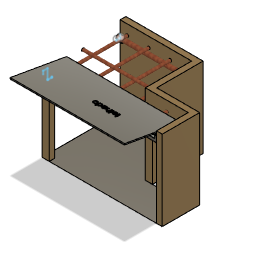
pergolado (Autodesk Fusion 360 design; units mm, degrees)
Autodesk Fusion 360 part; units mm, degrees
note: some values were not read from the file. Set by a fixed rule: which sketch regions a step uses.
sketch "Sketch1" plane through (0, 0, 0) normal (0, 1, 0) x (1, 0, 0)
  line L0 (0, 0) -> (2500, 0)
  line L1 (4000, -1620) -> (4000, -2730)
  line L2 (4000, -2730) -> (0, -2730)
  line L3 (0, -2730) -> (0, 0)
  line L4 (2500, 0) -> (2500, -1620)
  line L5 (2500, -1620) -> (4000, -1620)
  line L6 (0, -2730) -> (250, -2730)
  line L7 (250, -2730) -> (250, -2540)
  line L8 (250, -2540) -> (0, -2540)
  line L9 (0, -2540) -> (0, -2730)
  line L10 (0, 0) -> (2500, 0)
  line L11 (2500, 200) -> (0, 200)
  line L12 (0, 200) -> (0, 0)
  line L13 (2500, 200) -> (2700, 200)
  line L14 (2700, 200) -> (2700, -1420)
  line L15 (2700, -1620) -> (2500, -1620)
  line L16 (2500, -1620) -> (2500, 0)
  line L17 (2500, -1620) -> (4000, -1620)
  line L18 (4000, -1420) -> (2700, -1420)
  line L19 (2500, -1420) -> (2500, -1620)
  line L20 (4000, -1420) -> (4200, -1420)
  line L21 (4200, -1420) -> (4200, -2730)
  line L22 (4200, -2730) -> (4000, -2730)
  line L23 (4000, -2730) -> (4000, -1620)
  dimension "d2" = 2730
  dimension "d5" = 250
  dimension "d6" = 190
  dimension "d11" = 200
  dimension "d12" = 200
  dimension "d13" = 200
  dimension "d14" = 200
  constraint horizontal L0
  constraint vertical L1
  constraint horizontal L2
  constraint vertical L3
  constraint coincident L0.start L3.end
  constraint vertical L4
  constraint horizontal L5
  constraint horizontal L6
  constraint vertical L7
  constraint horizontal L8
  constraint vertical L9
  constraint horizontal L10
  constraint horizontal L11
  constraint vertical L12
  constraint horizontal L13
  constraint vertical L14
  constraint horizontal L15
  constraint vertical L16
  constraint horizontal L17
  constraint horizontal L18
  constraint vertical L19
  constraint horizontal L20
  constraint vertical L21
  constraint horizontal L22
  constraint vertical L23
  measures "d2" distance of L0.start L2.end
  measures "d5" distance of L2.end L6.end
  measures "d6" distance of L2.end L8.end
  measures "d11" distance of L0.start L11.end
  measures "d12" distance of L11.start L13.end
  measures "d13" distance of L4.end L19.start
  measures "d14" distance of L18.start L20.end
extrude "Extrude3" add sketch "Sketch1" along normal blind 2800 contours L0 L1 L4 L5 L10 L11 L12 L13 L14 L15 L16 L17 L18 L19 L20 L21 L22 L23 makes body 1
extrude "Extrude2" add sketch "Sketch1" against normal blind 1 separate body contours L0 L1 L2 L3 L4 L5 L7 L8 L10 L15 L16 L17 L19 L23 makes body 2
extrude "Extrude1" add sketch "Sketch1" along normal blind 2400 separate body contours L2 L3 L6 L7 L8 L9 makes body 3
sketch "Sketch2" plane through (0, 2400, 0) normal (0, 1, 0) x (-1, 0, 0)
  line L0 (0, 2540) -> (0, 2730)
  line L1 (0, 2730) -> (-250, 2730)
  line L2 (-250, 2730) -> (-250, 2540)
  line L3 (-250, 2540) -> (0, 2540)
  line L4 (0, 2540) -> (-4000, 2540)
  line L5 (-4000, 2540) -> (-4000, 2690)
  line L6 (-4000, 2690) -> (0, 2690)
  line L7 (0, 2690) -> (0, 2540)
  dimension "d17" = 4000
  dimension "d18" = 150
  constraint horizontal L4
  constraint vertical L5
  constraint horizontal L6
  constraint vertical L7
  constraint coincident L0.start L3.end
  measures "d17" distance of L0.start L4.end
  measures "d18" distance of L0.start L6.end
extrude "Extrude4" add sketch "Sketch2" along normal blind 200 separate body contours L0 L2 L3 L4 L6 L7 | L2 L4 L5 L6 makes body 4
sketch "Sketch3" plane through (0, 0, 0) normal (1, 0, 0) x (0, 0, -1)
  line L0 (-2540, 2600) -> (-2490, 2600) construction
  line L1 (-1890, 2536.1588) -> (-1890, 2485.3875)
  line L2 (-2531.3176, 2649.2404) -> (-1890, 2536.1588)
  line L3 (-2531.3176, 2649.2404) -> (-3516.1253, 2822.8886)
  line L4 (-2540, 2600) -> (-3524.8078, 2773.6482)
  line L5 (-2540, 2600) -> (-1890, 2485.3875)
  line L6 (-3516.1253, 2822.8886) -> (-3524.8078, 2773.6482)
  line L7 (-1890, 2536.1588) -> (-1881.3176, 2585.3992)
  line L8 (-1890, 2536.1588) -> (-1840, 2536.1588) construction
  line L9 (-1881.3176, 2585.3992) -> (-1930.558, 2594.0816)
  line L10 (-1930.558, 2594.0816) -> (-1939.2404, 2544.8412)
  dimension "d22" = 50
  dimension "d25" = 1000
  dimension "d26" = 1000
  dimension "d29" = 80
  dimension "d30" = 50
  dimension "d31" = 50
  constraint horizontal L0
  constraint perpendicular L4 L6
  constraint horizontal L8
  constraint perpendicular L2 L7
  constraint perpendicular L7 L9
  constraint coincident L2 L10.end
  constraint perpendicular L2 L10
  measures "d22" distance of L0.start L2.start
  measures "d25" distance of L2.start L3.end
  measures "d26" distance of L0.start L4.end
  measures "d29" angle of L7 L8
  measures "d30" distance of L1.start L7.end
  measures "d31" distance of L7.end L9.end
extrude "Extrude6" add sketch "Sketch3" along normal blind 4000 separate body contours L2 L7 L9 L10 makes body 5
extrude "Extrude5" add sketch "Sketch3" along normal blind 50 separate body contours L1 L2 L3 L4 L5 L6 makes body 6
copy_body "CopyPasteBodies1" bodies 6 makes body 7
move_body "Move1" bodies 7 to x (1, 0, 0) y (0, 1, 0) z (0, 0, 1) at (500, 0, 0)
copy_body "CopyPasteBodies2" bodies 6 makes body 8
move_body "Move2" bodies 8 to x (1, 0, 0) y (0, 1, 0) z (0, 0, 1) at (1000, 0, 0)
copy_body "CopyPasteBodies3" bodies 6 7 8 makes body 9 makes body 10 makes body 11
copy_body "CopyPasteBodies4" bodies 6 7 8 makes body 12 makes body 13 makes body 14
move_body "Move3" bodies 12 13 14 to x (1, 0, 0) y (0, 1, 0) z (0, 0, 1) at (1500, 0, 0)
copy_body "CopyPasteBodies6" bodies 6 7 8 makes body 15 makes body 16 makes body 17
copy_body "CopyPasteBodies7" bodies 14 13 makes body 18 makes body 19
move_body "Move5" bodies 18 19 to x (1, 0, 0) y (0, 1, 0) z (0, 0, 1) at (1000, 0, 0)
copy_body "CopyPasteBodies12" bodies 5 makes body 20
move_body "Move6" bodies 20 to x (1, 0, 0) y (0, 1, 0) z (0, 0, 1) at (0, 50.692, 289.2289)
copy_body "CopyPasteBodies13" bodies 20 5 makes body 21 makes body 22
move_body "Move7" bodies 21 22 to x (1, 0, 0) y (0, 1, 0) z (0, 0, 1) at (0, 91.3858, 516.4822)
sketch "Sketch4" plane through (0, 0, 0) normal (1, 0, 0) x (0, 0, -1)
  line L0 (0, 2325) -> (-2500, 2325)
  circle A0 centre (-79.8401, 2325) radius 75
  circle A1 centre (-1706.5871, 2325) radius 75
  circle A2 centre (-2458.2817, 2325) radius 75
  dimension "d35" = 150
  dimension "d36" = 150
  dimension "d37" = 150
  constraint coincident L0 A0.centre
  constraint coincident L0 A1.centre
  constraint coincident L0 A2.centre
  measures "d35" diameter of A0
  measures "d36" diameter of A1
  measures "d37" diameter of A2
extrude "Extrude8" add sketch "Sketch4" along normal blind 2500 separate body contours L0 A0 | L0 A0 makes body 23
extrude "Extrude7" add sketch "Sketch4" along normal blind 4000 separate body contours A2 makes body 24
extrude "Extrude9" add sketch "Sketch4" along normal blind 1500 separate body contours L0 A1 | L0 A1 makes body 25
move_body "Move8" bodies 25 to x (1, 0, 0) y (0, 1, 0) z (0, 0, 1) at (2500, 0, 0)
sketch "Sketch5" plane through (0, 0, 0) normal (0, 0, 1) x (1, 0, 0)
  line L0 (4000, 2400) -> (3250, 2400)
  line L1 (3250, 2400) -> (3250, 2450)
  circle A0 centre (3250, 2450) radius 50
  line L2 (2445.0116, 2400) -> (2445, 2450)
  circle A1 centre (2445, 2450) radius 50
  line L3 (3194.9659, 2408.2764) -> (2445.0116, 2400)
  line L4 (1750, 2400) -> (1750, 2450)
  circle A2 centre (1000, 2450) radius 50
  line L5 (1750, 2400) -> (1000, 2400)
  circle A3 centre (1750, 2450) radius 50
  line L6 (1000, 2400) -> (1000, 2450)
  line L7 (2500, 2400) -> (1750, 2400)
  line L8 (1000, 2400) -> (250, 2400)
  line L9 (250, 2400) -> (250, 2450)
  circle A4 centre (250, 2450) radius 50
  dimension "d48" = 750
  dimension "d49" = 50
  dimension "d50" = 100
  dimension "d51" = 750
  dimension "d52" = 50
  dimension "d53" = 100
  dimension "d54" = 750
  dimension "d55" = 50
  dimension "d56" = 100
  dimension "d57" = 750
  dimension "d58" = 50
  dimension "d59" = 100
  dimension "d60" = 750
  dimension "d61" = 50
  dimension "d62" = 100
  constraint coincident L1.end A0.centre
  constraint coincident L2.end A1.centre
  constraint coincident L4.end A3.centre
  constraint coincident A2.centre L6.end
  constraint coincident L9.end A4.centre
  measures "d48" distance of L0.start L0.end
  measures "d49" distance of L0.end L1.end
  measures "d50" diameter of A0
  measures "d51" distance of L2.start L3.start
  measures "d52" distance of L2.start L2.end
  measures "d53" diameter of A1
  measures "d54" distance of L4.start L7.start
  measures "d55" distance of L4.start L4.end
  measures "d56" diameter of A3
  measures "d57" distance of L5.end L4.start
  measures "d58" distance of L5.end A2.centre
  measures "d59" diameter of A2
  measures "d60" distance of L8.end L5.end
  measures "d61" distance of L8.end L9.end
  measures "d62" diameter of A4
extrude "Extrude15" add sketch "Sketch5" along normal blind 2600 separate body contours A1 | A2 | A3 | A4 makes body 26 at (1046.9846, 2467.101, 866.6667) makes body 27 at (1703.9262, 2430.5783, 866.6667) makes body 28 at (296.9846, 2467.101, 866.6667) makes body 29 at (2411.9157, 2487.4891, 1733.3333)
extrude "Extrude16" add sketch "Sketch5" along normal blind 1000 separate body contours A0 makes body 30
move_body "Move10" bodies 30 to x (1, 0, 0) y (0, 1, 0) z (0, 0, 1) at (0, 0, 1600)
sketch "Sketch7" plane through (0, 0, 0) normal (1, 0, 0) x (0, 0, -1)
  line L0 (0, 2500) -> (-1300, 2500)
  line L1 (-1300, 2500) -> (-1300, 2550)
  circle A0 centre (-1300, 2550) radius 50
  dimension "d77" = 50
  dimension "d78" = 100
  constraint horizontal L0
  constraint perpendicular L0 L1
  constraint coincident L1.end A0.centre
  measures "d77" distance of L0.end L1.end
  measures "d78" diameter of A0
extrude "Extrude17" add sketch "Sketch7" along normal blind 2500 separate body makes body 31
sketch "Sketch8" plane through (0, 0, 0) normal (1, 0, 0) x (0, 0, -1)
  line L0 (-1930.5, 2594) -> (-1890.5, 2594) construction
  line L1 (-1881.3178, 2585.3988) -> (-1874.3719, 2624.7911)
  line L2 (-1881.3178, 2585.3988) -> (-1841.3178, 2585.3988) construction
  line L3 (-1874.3719, 2624.7911) -> (-3843.9874, 2972.0875)
  line L4 (-1874.3719, 2624.7911) -> (125.6281, 2624.7911) construction
  line L5 (-1881.3178, 2585.3988) -> (-3850.9334, 2932.6952)
  line L6 (-3843.9874, 2972.0875) -> (-3850.9334, 2932.6952)
  dimension "d84" = 80
  dimension "d85" = 40
  dimension "d86" = 170
  dimension "d87" = 2000
  dimension "d88" = 2000
  constraint horizontal L0
  constraint horizontal L2
  constraint horizontal L4
  constraint perpendicular L5 L6
  measures "d84" angle of L1 L2
  measures "d85" distance of L1.start L1.end
  measures "d86" angle of L3 L4
  measures "d87" distance of L1.end L3.end
  measures "d88" distance of L1.start L5.end
extrude "Extrude18" add sketch "Sketch8" along normal blind 4000 separate body makes body 32
sketch "Sketch9" plane through (0, 2225.1075, -392.3465) normal (0, 0.984808, -0.173648) x (-1, 0, 0)
  line L0 (0, 2301.6862) -> (0, 4301.6862)
  line L1 (0, 4301.6862) -> (-4000, 4301.6862)
  line L2 (-4000, 4301.6862) -> (-4000, 2301.6862)
  line L3 (-4000, 2301.6862) -> (0, 2301.6862)
  line L4 (-2900, 3000) -> (-1400, 3000) construction
  line L5 (-1400, 3000) -> (-1400, 3500) construction
  line L6 (-1400, 3500) -> (-2900, 3500) construction
  line L7 (-2900, 3500) -> (-2900, 3000) construction
  dimension "d91" = 200
  text T0 "telhado" font "Arial" height 200 align left top in box 1500 x 500 at (-2900, 3000) x (1, 0) y (0, 1) spacing 1
extrude "Extrude19" cut sketch "Sketch9" against normal blind 10 text T0 bodies 32
sketch "Sketch10" plane through (0, 0, 1620) normal (0, 0, 1) x (1, 0, 0)
  line L0 (2500, 0) -> (4000, 0)
  line L1 (4000, 0) -> (4000, 2800)
  line L2 (4000, 2800) -> (2500, 2800)
  line L3 (2500, 2800) -> (2500, 0)
  line L4 (4000, 0) -> (3750, 0)
  line L5 (3750, 0) -> (3750, 2200)
  line L6 (3750, 2200) -> (2750, 2200)
  line L7 (2750, 2200) -> (2750, 0)
  line L8 (2750, 0) -> (4000, 0)
  dimension "d94" = 250
  dimension "d95" = 2200
  dimension "d96" = 1000
  dimension "d97" = 2200
  constraint coincident L0.end L1.start
  constraint perpendicular L3 L4
  constraint perpendicular L4 L5
  constraint perpendicular L5 L6
  constraint perpendicular L6 L7
  measures "d94" distance of L0.end L4.end
  measures "d95" distance of L4.end L5.end
  measures "d96" distance of L5.end L6.end
  measures "d97" distance of L6.end L7.end
extrude "Extrude20" cut sketch "Sketch10" against normal blind 500 contours L0 L5 L6 L7 L8 bodies 1
sketch "Sketch11" plane through (0, 0, 0) normal (1, 0, 0) x (0, 0, -1)
  line L0 (-2690.5, 2600) -> (-2539.5, 2600)
  line L1 (-2692.5, 2600) -> (-2692.5, 2500)
  line L2 (-2692.5, 2500) -> (-2690.5, 2500)
  line L3 (-2690.5, 2500) -> (-2690.5, 2600)
  line L4 (-2692.5, 2600) -> (-2692.5, 2602)
  line L5 (-2692.5, 2602) -> (-2537.5, 2602)
  line L6 (-2537.5, 2602) -> (-2537.5, 2600)
  line L7 (-2387.5, 2270) -> (-2385.5, 2270)
  line L8 (-2385.5, 2270) -> (-2385.5, 2248)
  line L9 (-2385.5, 2248) -> (-2539.5, 2248)
  line L10 (-2539.5, 2248) -> (-2539.5, 2600)
  line L11 (-2537.5, 2250) -> (-2520, 2250)
  line L12 (-2520, 2250) -> (-2537.5, 2267.5)
  line L13 (-2518, 2250) -> (-2537.5, 2269.5)
  line L14 (-2387.5, 2250) -> (-2400, 2250)
  line L15 (-2400, 2250) -> (-2387.5, 2262.5)
  line L16 (-2402, 2250) -> (-2387.5, 2264.5)
  line L17 (-2387.5, 2250) -> (-2387.5, 2262.5)
  line L18 (-2387.5, 2264.5) -> (-2387.5, 2270)
  line L19 (-2400, 2250) -> (-2387.5, 2250)
  line L20 (-2537.5, 2600) -> (-2537.5, 2269.5)
  line L21 (-2537.5, 2267.5) -> (-2537.5, 2250)
  line L22 (-2537.5, 2250) -> (-2520, 2250)
  line L23 (-2518, 2250) -> (-2402, 2250)
  line L24 (0, 2250) -> (0, 2360)
  line L25 (0, 2360) -> (-2, 2360)
  line L26 (-2, 2248) -> (0, 2248)
  line L27 (0, 2248) -> (0, 2250)
  line L28 (-2, 2248) -> (-142, 2248)
  line L29 (-142, 2250) -> (-142, 2248)
  line L30 (-2, 2250) -> (-22, 2250)
  line L31 (-22, 2250) -> (-2, 2270)
  line L32 (-22, 2250) -> (6.2843, 2250) construction
  line L33 (-2, 2272) -> (-24, 2250)
  line L34 (-2, 2272) -> (29.1127, 2272) construction
  line L35 (-142, 2250) -> (-142, 2270)
  line L36 (-142, 2270) -> (-140, 2270)
  line L37 (-140, 2268) -> (-140, 2250)
  line L38 (-140, 2270) -> (-120, 2250)
  line L39 (-140, 2270) -> (-111.7157, 2270) construction
  line L40 (-140, 2268) -> (-122, 2250)
  line L41 (-2, 2360) -> (-2, 2272)
  line L42 (-2, 2270) -> (-2, 2250)
  line L43 (-80, 2250) -> (-24, 2250)
  line L44 (-22, 2250) -> (-2, 2250)
  line L45 (-80, 2250) -> (-120, 2250)
  line L46 (-122, 2250) -> (-142, 2250)
  dimension "d101" = 155
  dimension "d102" = 100
  dimension "d103" = 2
  dimension "d104" = 2
  dimension "d105" = 155
  dimension "d106" = 180
  dimension "d107" = 350
  dimension "d108" = 150
  dimension "d109" = 2
  dimension "d110" = 22
  dimension "d111" = 154
  dimension "d112" = 45
  dimension "d113" = 2
  dimension "d114" = 2
  dimension "d115" = 45
  dimension "d116" = 2
  dimension "d117" = 2
  dimension "d124" = 2
  dimension "d125" = 90
  dimension "d126" = 2
  dimension "d127" = 90
  dimension "d128" = 140
  dimension "d129" = 20
  dimension "d130" = 45
  dimension "d131" = 2
  dimension "d132" = 135
  dimension "d133" = 20
  dimension "d134" = 2
  dimension "d135" = 45
  dimension "d136" = 2
  constraint horizontal L0
  constraint perpendicular L0 L1
  constraint perpendicular L1 L2
  constraint perpendicular L0 L3
  constraint perpendicular L0 L4
  constraint perpendicular L1 L5
  constraint perpendicular L20 L22
  constraint perpendicular L17 L22
  constraint perpendicular L7 L17
  constraint perpendicular L8 L22
  constraint perpendicular L9 L20
  constraint perpendicular L0 L10
  constraint perpendicular L11 L20
  constraint coincident L12.end L20
  constraint coincident L13.start L22
  constraint parallel L12 L13
  constraint coincident L14.end L22
  constraint coincident L16.end L17
  constraint parallel L15 L16
  constraint collinear L17 L18
  constraint collinear L19 L22
  constraint collinear L20 L21
  constraint collinear L22 L23
  constraint horizontal L43
  constraint perpendicular L24 L43
  constraint perpendicular L24 L25
  constraint perpendicular L27 L43
  constraint parallel L28 L45
  constraint perpendicular L29 L45
  constraint horizontal L32
  constraint coincident L31.end L41
  constraint horizontal L34
  constraint perpendicular L35 L45
  constraint perpendicular L35 L36
  constraint coincident L37.end L45
  constraint perpendicular L37 L45
  constraint horizontal L39
  constraint coincident L40.end L45
  constraint parallel L38 L40
  constraint collinear L41 L42
  constraint collinear L43 L44
  constraint collinear L45 L46
  measures "d101" distance of L1.start L6.end
  measures "d102" distance of L1.start L1.end
  measures "d103" distance of L1.end L2.end
  measures "d104" distance of L1.start L4.end
  measures "d105" distance of L4.end L5.end
  measures "d106" angle of L6 L20
  measures "d107" distance of L6.end L11.start
  measures "d108" distance of L11.start L14.start
  measures "d109" distance of L7.start L7.end
  measures "d110" distance of L7.end L8.end
  measures "d111" distance of L8.end L9.end
  measures "d112" angle of L11 L12
  measures "d113" distance of L12.end L13.end
  measures "d114" distance of L11.end L13.start
  measures "d115" angle of L14 L15
  measures "d116" distance of L15.end L16.end
  measures "d117" distance of L14.end L16.start
  measures "d124" distance of L24.end L25.end
  measures "d125" angle of L25 L41
  measures "d126" distance of L30.start L26.start
  measures "d127" angle of L27 L28
  measures "d128" distance of L26.start L28.end
  measures "d129" distance of L30.start L30.end
  measures "d130" angle of L31 L32
  measures "d131" distance of L31.end L33.start
  measures "d132" angle of L33 L34
  measures "d133" distance of L29.start L35.end
  measures "d134" distance of L35.end L36.end
  measures "d135" angle of L38 L39
  measures "d136" distance of L36.end L37.start
extrude "Extrude23" add sketch "Sketch11" along normal blind 200 separate body contours L24 L25 L26 L27 L28 L29 L33 L35 L36 L38 L41 L43 L45 makes body 33
extrude "Extrude21" add sketch "Sketch11" along normal blind 200 separate body contours L0 L1 L2 L3 L4 L5 L6 L7 L8 L9 L10 L13 L16 L18 L20 L23 makes body 34
sketch "Sketch12" plane through (0, 2248, 0) normal (0, -1, 0) x (1, 0, 0)
  line L0 (0, 2539.5) -> (0, 2385.5)
  line L1 (0, 2385.5) -> (200, 2385.5)
  line L2 (200, 2385.5) -> (200, 2539.5)
  line L3 (200, 2539.5) -> (0, 2539.5)
  line L4 (0, 2539.5) -> (200, 2539.5)
  line L5 (200, 2539.5) -> (200, 2385.5)
  line L6 (200, 2385.5) -> (0, 2385.5)
  line L7 (0, 2385.5) -> (0, 2539.5)
  circle A0 centre (100, 2460) radius 5
  dimension "d120" = 10
  constraint horizontal L4
  constraint vertical L5
  constraint horizontal L6
  constraint vertical L7
  constraint coincident L1.end L2.start
  constraint coincident L0.start L3.end
  measures "d120" diameter of A0
extrude "Extrude22" cut sketch "Sketch12" against normal blind 2 contours A0 bodies 34
copy_body "CopyPasteBodies15" bodies 34 makes body 35
move_body "Move12" bodies 35 to x (1, 0, 0) y (0, 1, 0) z (0, 0, 1) at (3700, 0, 0)
move_body "Move13" bodies 23 to x (1, 0, 0) y (0, 1, 0) z (0, 0, 1) at (0, 0, -2)
sketch "Sketch13" plane through (0, 2248, 0) normal (0, -1, 0) x (1, 0, 0)
  line L0 (0, 142) -> (0, 0)
  line L1 (0, 0) -> (200, 0)
  line L2 (200, 0) -> (200, 142)
  line L3 (200, 142) -> (0, 142)
  line L4 (0, 142) -> (200, 142)
  line L5 (200, 142) -> (200, 0)
  line L6 (200, 0) -> (0, 0)
  line L7 (0, 0) -> (0, 142)
  circle A0 centre (100, 71) radius 5
  dimension "d139" = 10
  constraint horizontal L4
  constraint vertical L5
  constraint horizontal L6
  constraint vertical L7
  constraint coincident L1.end L2.start
  constraint coincident L0.start L3.end
  measures "d139" diameter of A0
extrude "Extrude24" cut sketch "Sketch13" against normal blind 2 contours A0 bodies 33
sketch "Sketch14" plane through (0, 0, 2) normal (0, 0, 1) x (1, 0, 0)
  line L0 (0, 2360) -> (0, 2272)
  line L1 (0, 2272) -> (200, 2272)
  line L2 (200, 2272) -> (200, 2360)
  line L3 (200, 2360) -> (0, 2360)
  line L4 (0, 2360) -> (200, 2360)
  line L5 (200, 2360) -> (200, 2272)
  line L6 (200, 2272) -> (0, 2272)
  line L7 (0, 2272) -> (0, 2360)
  circle A0 centre (100, 2286) radius 5
  circle A1 centre (30, 2330) radius 5
  circle A2 centre (170.1133, 2330) radius 5
  line L8 (0, 2360) -> (0, 2330)
  line L9 (0, 2330) -> (30, 2330)
  line L10 (200, 2360) -> (200, 2330)
  line L11 (200, 2330) -> (170, 2330)
  dimension "d142" = 10
  dimension "d143" = 10
  dimension "d144" = 10
  dimension "d145" = 30
  dimension "d146" = 30
  constraint horizontal L4
  constraint vertical L5
  constraint horizontal L6
  constraint vertical L7
  constraint coincident L1.end L2.start
  constraint coincident L0.start L3.end
  constraint coincident L7 L8.end
  constraint perpendicular L3 L8
  constraint perpendicular L7 L9
  constraint perpendicular L3 L10
  constraint perpendicular L10 L11
  measures "d142" diameter of A0
  measures "d143" diameter of A1
  measures "d144" diameter of A2
  measures "d145" distance of L2.end L10.end
  measures "d146" distance of L10.end L11.end
extrude "Extrude25" cut sketch "Sketch14" against normal blind 2 contours A0 | A1 | A2 bodies 33
copy_body "CopyPasteBodies16" bodies 33 makes body 36
move_body "Move14" bodies 36 to x (1, 0, 0) y (0, 1, 0) z (0, 0, 1) at (2175, 0, 0)
extrude "Extrude10" [suppressed]
move_body "Move9" [suppressed]
extrude "Extrude11" [suppressed]
extrude "Extrude12" [suppressed]
extrude "Extrude13" [suppressed]
extrude "Extrude14" [suppressed]
named bodies: "pilastra", "Piso", "muro", "Viga metal", "apoio telhado", "Fim telhado", "apoio telhado (1)", "apoio telhado (1) (1)", "apoio telhado (2)", "apoio telhado (1) (1) (1)", "apoio telhado (1) (1) (1) (1)", "apoio telhado (3)", "apoio telhado (1) (2)", "apoio telhado (1) (1) (2)", "apoio telhado (4)", "apoio telhado (1) (3)", "apoio telhado (1) (1) (3)", "apoio telhado (1) (1) (2) (1)", "apoio telhado (1) (2) (1)", "Fim telhado (1)", "Fim telhado (2)", "Fim telhado (1) (1)", "telhado (1)", "suporte viga", "suporte viga (1)"
